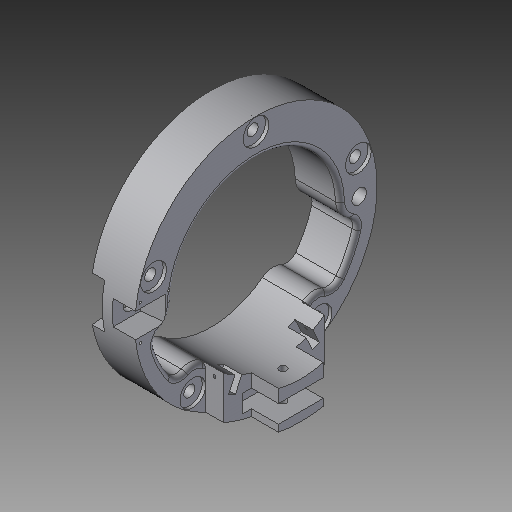
# Autodesk Inventor part: 3218_Coil Holder End_V1
Saved by Autodesk Inventor 2020 (Build 240168000, 168)
## iProperties
Created: 2018-08-02
Part Number: 3218_Coil Holder End_V1
Material: Acetal Resin, White
Document SubType Name: Modeling
Designer: em364
Density: 1.425 g/cm^3
Appearance: Smooth - White
Mass: 120.541 g
Surface Area: 258.548 cm^2
Volume: 84.5901 cm^3
Author: em364
Autodesk Inventor part; units mm, degrees
sketch "Sketch1" plane through (0, 0, 0) normal (1, 0, 0) x (0, 1, 0)
  circle A0 centre (0, 0) radius 54
  circle A1 centre (0, 46) radius 3.25
  circle A2 centre (0, -46) radius 3.25
  circle A3 centre (0, 0) radius 37.5
  circle A4 centre (48, 0) radius 2.5
  circle A5 centre (14.8328, 45.6507) radius 2.5
  circle A6 centre (-38.8328, 28.2137) radius 2.5
  circle A7 centre (-38.8328, -28.2137) radius 2.5
  circle A8 centre (14.8328, -45.6507) radius 2.5
  dimension "d0" = 108
  dimension "d4" = 6.5
  dimension "d5" = 6.5
  dimension "d67" = 75
  dimension "d71" = 0
  dimension "d72" = 0
  dimension "d73" = 46
  dimension "d74" = 46
  dimension "d76" = 5
  dimension "d77" = 48
  dimension "d80" = 360
  constraints: 9 centre point, 11 other
  measures "d0" diameter of A0
  measures "d4" diameter of A2
  measures "d5" diameter of A1
  measures "d67" diameter of A3
  measures "d71" distance of A0.centre A3.centre
  measures "d72" distance of A0.centre A3.centre
  measures "d73" distance of A0.centre A1.centre
  measures "d74" distance of A0.centre A2.centre
  measures "d76" diameter of A4
  measures "d77" distance of A0.centre A4.centre
extrude "Extrusion5" add sketch "Sketch1" along normal blind 20
sketch "Sketch5" plane through (20, 0, 0) normal (1, 0, 0) x (0, 0, -1)
  circle A0 centre (0, 0) radius 37.5 projected
  circle A1 centre (46, 0) radius 3.25 projected
  circle A2 centre (-46, 0) radius 3.25 projected
  circle A3 centre (45.6507, 14.8328) radius 2.5 projected
  circle A4 centre (28.2137, -38.8328) radius 2.5 projected
  circle A5 centre (-28.2137, -38.8328) radius 2.5 projected
  circle A6 centre (-45.6507, 14.8328) radius 2.5 projected
  circle A7 centre (0, 48) radius 2.5 projected
  circle A8 centre (0, 0) radius 54 projected
  circle A9 centre (0, 48) radius 5.75
  circle A10 centre (0, 48) radius 2.5 projected
  circle A11 centre (-45.6507, 14.8328) radius 5.75
  circle A12 centre (-28.2137, -38.8328) radius 5.75
  circle A13 centre (28.2137, -38.8328) radius 5.75
  circle A14 centre (45.6507, 14.8328) radius 5.75
  dimension "d84" = 11.5
  dimension "d87" = 360
  constraints: 5 centre point, 1 coincident, 1 concentric, 11 other
  measures "d84" diameter of A9
extrude "Extrusion6" cut sketch "Sketch5" against normal blind 1.5 contours A9 | A11 | A12 | A13 | A14
sketch "Sketch6" plane through (0, 0, 0) normal (-1, 0, 0) x (0, 0, 1)
  circle A0 centre (0, 0) radius 42 construction
  line L0 (0, 0) -> (20.2657, 62.3715) construction
  circle A1 centre (0, 48) radius 2.5 projected
  line L1 (0, 48) -> (0, 0) construction
  line L2 (10.0924, 40.7694) -> (13.808, 52.2048)
  circle A2 centre (0, 0) radius 54 projected
  line L3 (15.7987, 38.9153) -> (19.5143, 50.3507)
  arc A3 (15.7987, 38.9153) -> (10.0924, 40.7694) centre (0, 0) ccw
  arc A4 (19.5143, 50.3507) -> (13.808, 52.2048) centre (0, 0) ccw
  line L4 (-15.7987, 38.9153) -> (-19.5143, 50.3507)
  line L5 (-10.0924, 40.7694) -> (-13.808, 52.2048)
  arc A5 (-10.0924, 40.7694) -> (-15.7987, 38.9153) centre (0, 0) ccw
  arc A6 (-13.808, 52.2048) -> (-19.5143, 50.3507) centre (0, 0) ccw
  line L6 (-35.6553, 22.1969) -> (-45.3828, 29.2643)
  line L7 (-32.1286, 27.051) -> (-41.8561, 34.1184)
  arc A7 (-32.1286, 27.051) -> (-35.6553, 22.1969) centre (0, 0) ccw
  arc A8 (-41.8561, 34.1184) -> (-45.3828, 29.2643) centre (0, 0) ccw
  line L8 (-41.8927, -3) -> (-53.9166, -3)
  line L9 (-41.8927, 3) -> (-53.9166, 3)
  arc A9 (-41.8927, 3) -> (-41.8927, -3) centre (0, 0) ccw
  arc A10 (-53.9166, 3) -> (-53.9166, -3) centre (0, 0) ccw
  line L10 (-32.1286, -27.051) -> (-41.8561, -34.1184)
  line L11 (-35.6553, -22.1969) -> (-45.3828, -29.2643)
  arc A11 (-35.6553, -22.1969) -> (-32.1286, -27.051) centre (0, 0) ccw
  arc A12 (-45.3828, -29.2643) -> (-41.8561, -34.1184) centre (0, 0) ccw
  line L12 (-10.0924, -40.7694) -> (-13.808, -52.2048)
  line L13 (-15.7987, -38.9153) -> (-19.5143, -50.3507)
  arc A13 (-15.7987, -38.9153) -> (-10.0924, -40.7694) centre (0, 0) ccw
  arc A14 (-19.5143, -50.3507) -> (-13.808, -52.2048) centre (0, 0) ccw
  line L14 (15.7987, -38.9153) -> (19.5143, -50.3507)
  line L15 (10.0924, -40.7694) -> (13.808, -52.2048)
  arc A15 (10.0924, -40.7694) -> (15.7987, -38.9153) centre (0, 0) ccw
  arc A16 (13.808, -52.2048) -> (19.5143, -50.3507) centre (0, 0) ccw
  line L16 (35.6553, -22.1969) -> (45.3828, -29.2643)
  line L17 (32.1286, -27.051) -> (41.8561, -34.1184)
  arc A17 (32.1286, -27.051) -> (35.6553, -22.1969) centre (0, 0) ccw
  arc A18 (41.8561, -34.1184) -> (45.3828, -29.2643) centre (0, 0) ccw
  line L18 (41.8927, 3) -> (53.9166, 3)
  line L19 (41.8927, -3) -> (53.9166, -3)
  arc A19 (41.8927, -3) -> (41.8927, 3) centre (0, 0) ccw
  arc A20 (53.9166, -3) -> (53.9166, 3) centre (0, 0) ccw
  line L20 (32.1286, 27.051) -> (41.8561, 34.1184)
  line L21 (35.6553, 22.1969) -> (45.3828, 29.2643)
  arc A21 (35.6553, 22.1969) -> (32.1286, 27.051) centre (0, 0) ccw
  arc A22 (45.3828, 29.2643) -> (41.8561, 34.1184) centre (0, 0) ccw
  line L22 (-12.9787, 39.9444) -> (0, 0) construction
  line L23 (0, 0) -> (-33.9787, 24.687) construction
  line L24 (0, 0) -> (-33.9787, -24.687) construction
  line L25 (0, 0) -> (-12.9787, -39.9444) construction
  line L26 (0, 0) -> (12.9787, -39.9444) construction
  line L27 (0, 0) -> (33.9787, -24.687) construction
  line L28 (0, 0) -> (33.9787, 24.687) construction
  line L29 (0, 0) -> (59.5549, -8.3699) construction
  line L30 (0, 0) -> (54, 0) construction
  line L31 (41.9025, -2.8595) -> (53.8094, -4.5329)
  line L32 (52.9744, -10.4745) -> (41.0675, -8.8011)
  arc A23 (41.0675, -8.8011) -> (41.9025, -2.8595) centre (0, 0) ccw
  arc A24 (52.9744, -10.4745) -> (53.8094, -4.5329) centre (0, 0) ccw
  line L33 (-41.8927, -3) -> (-53.9166, -3)
  line L34 (-41.9025, -2.8595) -> (-53.8094, -4.5329)
  line L35 (-52.9744, -10.4745) -> (-41.0675, -8.8011)
  arc A25 (-41.9025, -2.8595) -> (-41.0675, -8.8011) centre (0, 0) ccw
  arc A26 (-53.8094, -4.5329) -> (-52.9744, -10.4745) centre (0, 0) ccw
  line L36 (-41.5913, -5.8453) -> (0, 0) construction
  dimension "d91" = 84
  dimension "d92" = 18
  dimension "d93" = 3
  dimension "d94" = 3
  dimension "d97" = 360
  dimension "d99" = 18
  dimension "d100" = 54
  dimension "d101" = 54
  dimension "d102" = 18
  dimension "d103" = 18
  dimension "d104" = 54
  dimension "d105" = 54
  dimension "d106" = 8
  dimension "d107" = 3
  dimension "d108" = 3
  dimension "d109" = 8
  constraints: 74 end point, 65 point on circle, 25 centre point, 15 coincident, 4 parallel, 4 symmetric about line, 1 vertical, 103 other
  measures "d91" diameter of A0
  measures "d92" angle of L0 L1
  measures "d93" distance between parallel lines of L0 L2
  measures "d94" distance between parallel lines of L3 L0
  measures "d99" angle of L22 L1
  measures "d100" angle of L1 L23
  measures "d101" angle of L24 L1
  measures "d102" angle of L1 L25
  measures "d103" angle of L1 L26
  measures "d104" angle of L1 L27
  measures "d105" angle of L1 L28
  measures "d106" angle of L29 L30
  measures "d107" distance between parallel lines of L32 L29
  measures "d108" distance between parallel lines of L29 L31
  measures "d109" angle of L36 L30
extrude "Extrusion7" add sketch "Sketch6" along normal blind 100 contours L2 A2 L3 A3 | L5 A5 L4 A2 | A2 L21 A21 L20 | L7 A7 L6 A2 | L31 L19 A19 | A2 L32 A23 L19 L31 | L34 L8 A25 L35 A2 | L34 A9 L8 | A2 L17 A17 L16 | L11 A11 L10 A2 | A2 L15 A15 L14 | L13 A13 L12 A2
ref_plane "Work Plane4" through (-100, 0, 0) normal (-1, 0, 0) x (0, 0, 1)
sketch "Sketch7" plane through (-100, 0, 0) normal (-1, 0, 0) x (0, 0, 1)
  line L0 (45.3828, 29.2643) -> (35.6553, 22.1969) construction
  arc A0 (35.6553, 22.1969) -> (32.1286, 27.051) centre (0, 0) ccw projected
  line L1 (32.1286, 27.051) -> (41.8561, 34.1184) construction
  arc A1 (41.8561, 34.1184) -> (19.5143, 50.3507) centre (0, 0) ccw projected
  line L2 (19.5143, 50.3507) -> (15.7987, 38.9153) construction
  arc A2 (15.7987, 38.9153) -> (10.0924, 40.7694) centre (0, 0) ccw projected
  line L3 (10.0924, 40.7694) -> (13.808, 52.2048) construction
  arc A3 (13.808, 52.2048) -> (-13.808, 52.2048) centre (0, 0) ccw projected
  line L4 (-13.808, 52.2048) -> (-10.0924, 40.7694) construction
  arc A4 (-10.0924, 40.7694) -> (-15.7987, 38.9153) centre (0, 0) ccw projected
  line L5 (-15.7987, 38.9153) -> (-19.5143, 50.3507) construction
  arc A5 (-19.5143, 50.3507) -> (-41.8561, 34.1184) centre (0, 0) ccw projected
  line L6 (-41.8561, 34.1184) -> (-32.1286, 27.051) construction
  arc A6 (-32.1286, 27.051) -> (-35.6553, 22.1969) centre (0, 0) ccw projected
  line L7 (-35.6553, 22.1969) -> (-45.3828, 29.2643) construction
  arc A7 (-45.3828, 29.2643) -> (-53.8094, -4.5329) centre (0, 0) ccw projected
  line L8 (-53.8094, -4.5329) -> (-41.9025, -2.8595) construction
  arc A8 (-41.9025, -2.8595) -> (-41.0675, -8.8011) centre (0, 0) ccw projected
  line L9 (-41.0675, -8.8011) -> (-52.9744, -10.4745) construction
  arc A9 (-52.9744, -10.4745) -> (-45.3828, -29.2643) centre (0, 0) ccw projected
  line L10 (-45.3828, -29.2643) -> (-35.6553, -22.1969) construction
  arc A10 (-35.6553, -22.1969) -> (-32.1286, -27.051) centre (0, 0) ccw projected
  line L11 (-32.1286, -27.051) -> (-41.8561, -34.1184) construction
  arc A11 (-41.8561, -34.1184) -> (-19.5143, -50.3507) centre (0, 0) ccw projected
  line L12 (-19.5143, -50.3507) -> (-15.7987, -38.9153) construction
  arc A12 (-15.7987, -38.9153) -> (-10.0924, -40.7694) centre (0, 0) ccw projected
  line L13 (-10.0924, -40.7694) -> (-13.808, -52.2048) construction
  arc A13 (-13.808, -52.2048) -> (13.808, -52.2048) centre (0, 0) ccw projected
  line L14 (13.808, -52.2048) -> (10.0924, -40.7694) construction
  arc A14 (10.0924, -40.7694) -> (15.7987, -38.9153) centre (0, 0) ccw projected
  line L15 (15.7987, -38.9153) -> (19.5143, -50.3507) construction
  arc A15 (19.5143, -50.3507) -> (41.8561, -34.1184) centre (0, 0) ccw projected
  line L16 (41.8561, -34.1184) -> (32.1286, -27.051) construction
  arc A16 (32.1286, -27.051) -> (35.6553, -22.1969) centre (0, 0) ccw projected
  line L17 (35.6553, -22.1969) -> (45.3828, -29.2643) construction
  arc A17 (45.3828, -29.2643) -> (52.9744, -10.4745) centre (0, 0) ccw projected
  line L18 (52.9744, -10.4745) -> (41.0675, -8.8011) construction
  arc A18 (41.0675, -8.8011) -> (41.9025, -2.8595) centre (0, 0) ccw projected
  line L19 (41.9025, -2.8595) -> (53.8094, -4.5329) construction
  arc A19 (53.8094, -4.5329) -> (45.3828, 29.2643) centre (0, 0) ccw projected
  circle A20 centre (0, 48) radius 2.5 construction
  circle A21 centre (45.6507, 14.8328) radius 2.5 construction
  circle A22 centre (28.2137, -38.8328) radius 2.5 construction
  circle A23 centre (-28.2137, -38.8328) radius 2.5 construction
  circle A24 centre (-45.6507, 14.8328) radius 2.5 construction
  circle A25 centre (46, 0) radius 3.25 construction
  circle A26 centre (-46, 0) radius 3.25 projected
  circle A27 centre (0, 0) radius 37.5 projected
  circle A28 centre (0, 0) radius 54
  circle A29 centre (0, 0) radius 37.5 projected
  line L20 (0, 0) -> (0, -54) construction
  circle A30 centre (0, 0) radius 54 projected
  line L21 (0, 0) -> (-32.0095, -68.6446) construction
  circle A31 centre (0, 0) radius 42 construction
  line L22 (0, 0) -> (32.0095, -68.6446) construction
  line L23 (0, 0) -> (-46, 0) construction
  line L24 (0, 0) -> (-32.0095, 68.6446) construction
  line L25 (0, 0) -> (32.0095, 68.6446) construction
  arc A32 (-21.9138, 30.4308) -> (-21.9138, -30.4308) centre (0, 0) ccw
  arc A33 (9.2255, 36.3475) -> (-9.2255, 36.3475) centre (0, 0) ccw
  arc A34 (21.9138, -30.4308) -> (21.9138, 30.4308) centre (0, 0) ccw
  arc A35 (-9.2255, -36.3475) -> (9.2255, -36.3475) centre (0, 0) ccw
  circle A36 centre (0, 0) radius 37.5
  dimension "d113" = 25
  dimension "d115" = 84
  dimension "d120" = 25
  dimension "d123" = 25
  dimension "d124" = 25
  constraints: 12 end point, 11 point on circle, 9 symmetric about line, 7 centre point, 5 coincident, 1 concentric, 1 horizontal, 2 other
  measures "d113" angle of L21 L20
  measures "d115" diameter of A31
  measures "d120" angle of L20 L22
  measures "d123" angle of L20 L24
  measures "d124" angle of L20 L25
extrude "Extrusion12" add sketch "Sketch7" along normal blind 10
sketch "Sketch11" plane through (-110, 0, 0) normal (-1, 0, 0) x (0, 0, 1)
  circle A0 centre (0, 0) radius 37.5 projected
  circle A1 centre (-46, 0) radius 3.25 projected
  circle A2 centre (0, 0) radius 54 projected
  circle A3 centre (0, 0) radius 42 construction
  line L0 (0, 0) -> (-19.8631, 42.5965) construction
  arc A4 (-13.2974, 45.0797) -> (-25.9857, 39.1631) centre (0, 0) ccw projected
  line L1 (0, 0) -> (19.8631, 42.5965) construction
  arc A5 (25.9857, 39.1631) -> (13.2974, 45.0797) centre (0, 0) ccw projected
  line L2 (0, 0) -> (19.8631, -42.5965) construction
  arc A6 (13.2974, -45.0797) -> (25.9857, -39.1631) centre (0, 0) ccw projected
  arc A7 (37.5, 0) -> (37.5, 0) centre (0, 0) ccw projected
  line L3 (0, 0) -> (-19.8631, -42.5965) construction
  arc A8 (-25.9857, -39.1631) -> (-13.2974, -45.0797) centre (0, 0) ccw projected
  circle A9 centre (-17.75, 38.0649) radius 1.7
  circle A10 centre (17.75, 38.0649) radius 1.7
  circle A11 centre (17.75, -38.0649) radius 1.7
  circle A12 centre (-17.75, -38.0649) radius 1.7
  dimension "d151" = 84
  dimension "d152" = 3.4
  dimension "d153" = 3.4
  dimension "d154" = 3.4
  dimension "d155" = 3.4
  constraints: 8 end point, 8 point on circle, 5 centre point, 4 point on line, 1 coincident
  measures "d151" diameter of A3
  measures "d152" diameter of A9
  measures "d153" diameter of A10
  measures "d154" diameter of A11
  measures "d155" diameter of A12
extrude "Extrusion14" cut sketch "Sketch11" against normal blind 10 contours A9 | A10 | A11 | A12
ref_plane "Work Plane5" through (-50, 0, 0) normal (1, 0, 0) x (0, 0, -1)
sketch "Sketch12" plane through (-50, 0, 0) normal (1, 0, 0) x (0, 0, -1)
  circle A0 centre (45.6507, 14.8328) radius 5.75 construction
  circle A1 centre (-28.2137, -38.8328) radius 5.75 construction
  circle A2 centre (0, 48) radius 5.75 construction
  circle A3 centre (-45.6507, 14.8328) radius 5.75 construction
  circle A4 centre (28.2137, -38.8328) radius 5.75 construction
  circle A5 centre (0, 0) radius 37.5 projected
  circle A6 centre (46, 0) radius 3.25 projected
  circle A7 centre (-46, 0) radius 3.25 construction
  circle A8 centre (0, 0) radius 54 projected
extrude "Extrusion15" add sketch "Sketch12" along normal mid plane 6
sketch "Sketch13" plane through (20, 0, 0) normal (1, 0, 0) x (0, 0, -1)
  circle A0 centre (0, 0) radius 54 construction
  circle A1 centre (0, 0) radius 37.5 construction
  line L0 (0, 0) -> (0, -37.5)
  line L1 (0, 0) -> (60.8881, 0) construction
  line L2 (-22.5, -30) -> (-22.5, -49.0892)
  line L3 (22.5, -30) -> (22.5, -49.0892)
  arc A2 (-22.5, -30) -> (22.5, -30) centre (0, 0) ccw
  arc A3 (-22.5, -49.0892) -> (22.5, -49.0892) centre (0, 0) ccw
  dimension "d166" = 22.5
  dimension "d167" = 22.5
  constraints: 8 end point, 6 point on circle, 2 centre point, 2 coincident, 2 symmetric about line, 2 vertical, 1 horizontal, 2 other
  measures "d166" distance between parallel lines of L2 L0
  measures "d167" distance between parallel lines of L3 L0
extrude "Extrusion16" add sketch "Sketch13" along normal blind 8
sketch "Sketch14" plane through (28, 0, 0) normal (1, 0, 0) x (0, 0, -1)
  arc A0 (-22.5, -30) -> (22.5, -30) centre (0, 0) ccw projected
  line L0 (0, 0) -> (0, -37.5)
  circle A1 centre (0, 0) radius 54 projected
  line L1 (12, -42) -> (-12, -42) construction
  line L2 (-10, -42) -> (-10, -36.1421)
  line L3 (10, -42) -> (10, -36.1421)
  arc A2 (-10, -36.1421) -> (10, -36.1421) centre (0, 0) ccw
  line L4 (-10, -42) -> (10, -42)
  line L5 (-10, -50) -> (-10, -53.066)
  line L6 (10, -50) -> (10, -53.066)
  line L7 (-10, -50) -> (10, -50)
  arc A3 (-10, -53.066) -> (10, -53.066) centre (0, 0) ccw
  dimension "d174" = 16.5
  dimension "d194" = 10
  dimension "d195" = 10
  dimension "d196" = 8
  dimension "d197" = 10
  dimension "d198" = 10
  dimension "d211" = 50
  constraints: 16 end point, 5 point on circle, 4 symmetric about line, 2 centre point, 2 collinear, 1 coincident, 1 perpendicular, 1 point on line, 1 vertical
  measures "d174" radial gap between concentric circles of A1 A0
  measures "d194" distance between parallel lines of L0 L2
  measures "d195" distance between parallel lines of L0 L5
  measures "d196" distance between parallel lines of L7 L4
  measures "d197" distance between parallel lines of L0 L3
  measures "d198" distance between parallel lines of L0 L6
  measures "d211" distance from line of L7 point (0, 0)
extrude "Extrusion17" add sketch "Sketch14" along normal blind 12 contours A0 L3 L4 L2 | L5 L7 L6 A1 picked at (-1.1168, -51.2987)
sketch "Sketch16" plane through (28, 0, 0) normal (1, 0, 0) x (0, 0, -1)
  arc A0 (22.5, -49.0892) -> (-22.5, -49.0892) centre (0, 0) ccw projected
  line L0 (0, 0) -> (0, 37.5)
  circle A1 centre (0, 0) radius 37.5 construction
  line L1 (0, 0) -> (-18.722, -40.1494) construction
  line L2 (-18.722, -40.1494) -> (-17.1813, -40.8679)
  line L3 (-17.1813, -40.8679) -> (-14.2912, -34.6701)
  line L4 (-18.722, -40.1494) -> (-20.2627, -39.431)
  line L5 (-20.2627, -39.431) -> (-17.3726, -33.2331)
  line L6 (0, 0) -> (18.722, -40.1494) construction
  line L7 (18.722, -40.1494) -> (17.1813, -40.8679)
  line L8 (17.1813, -40.8679) -> (14.2912, -34.6701)
  line L9 (20.2627, -39.431) -> (17.3726, -33.2331)
  line L10 (18.722, -40.1494) -> (20.2627, -39.431)
  arc A2 (-17.3726, -33.2331) -> (-14.2912, -34.6701) centre (0, 0) ccw
  arc A3 (14.2912, -34.6701) -> (17.3726, -33.2331) centre (0, 0) ccw
  dimension "d187" = 25
  dimension "d188" = 44.3
  dimension "d190" = 1.7
  dimension "d212" = 44.3
  constraints: 22 end point, 7 symmetric about line, 6 point on circle, 2 centre point, 2 coincident, 2 perpendicular
  measures "d187" angle of L0 L1
  measures "d188" distance of L0.start L1.end
  measures "d190" distance of L1.end L2.end
  measures "d212" distance from line of L10 point (0, 0)
extrude "Extrusion19" cut sketch "Sketch16" against normal blind 8
ref_plane "Work Plane7" through (28, -32, -10) normal (0, -1, 0) x (1, 0, 0)
sketch "Sketch18" plane through (28, -32, -10) normal (0, -1, 0) x (1, 0, 0)
  line L0 (0, 20) -> (12, 20) construction
  line L1 (0, 0) -> (0, 20) construction
  line L2 (0, 0) -> (12, 0) construction
  line L3 (12, 20) -> (12, 0) construction
  circle A0 centre (4, 10) radius 1.65
  point P0 (-28, 10)
  dimension "d200" = 3.3
  dimension "d201" = 10
  dimension "d202" = 8
  dimension "d203" = 20
  constraints: 1 centre point
  measures "d200" diameter of A0
  measures "d201" distance from line of L0 A0.centre
  measures "d202" distance from line of A0.centre L3
  measures "d203" distance of L0.end L2.end
extrude "Extrusion20" cut sketch "Sketch18" along normal through all
sketch "Sketch19" plane through (-110, 0, 0) normal (-1, 0, 0) x (0, 0, 1)
  circle A0 centre (0, 0) radius 54 construction
  circle A1 centre (0, 0) radius 50 construction
  line L0 (-6.3, 50) -> (-6.3, 53.6312)
  arc A2 (13.808, 52.2048) -> (-13.808, 52.2048) centre (0, 0) ccw projected
  line L1 (0, 0) -> (0, 50) construction
  line L2 (0, 50) -> (6.1226, 50) construction
  line L3 (6.3, 50) -> (6.3, 53.6312)
  line L4 (0, 50) -> (-1.1865, 50) construction
  arc A3 (-6.3, 50) -> (6.3, 50) centre (0, 50) ccw
  circle A4 centre (0, 0) radius 54
  dimension "d206" = 100
  dimension "d208" = 50
  dimension "d213" = 6.3
  dimension "d215" = 0
  constraints: 10 end point, 6 point on circle, 3 coincident, 2 centre point, 2 horizontal, 2 vertical, 1 parallel, 1 point on line, 3 other
  measures "d206" diameter of A1
  measures "d208" distance of A1.centre L1.end
  measures "d213" radius of A3
  measures "d215" distance from line of L1 L4.start
extrude "Extrusion21" cut sketch "Sketch19" against normal up to surface (63 mm away) contours L0 A2 L3 A3
sketch "Sketch20" plane through (0, 0, 0) normal (-1, 0, 0) x (0, 0, 1)
  circle A0 centre (0, 0) radius 54
  constraints: 1 centre point, 1 coincident
extrude "Extrusion22" cut sketch "Sketch20" along normal through all
sketch "Sketch21" plane through (28, 0, 0) normal (1, 0, 0) x (0, 0, -1)
  line L0 (-14, -42) -> (14, -42)
  line L1 (14, -42) -> (14, -50)
  line L2 (14, -50) -> (-14, -50)
  line L3 (-14, -50) -> (-14, -42)
  line L4 (-10, -36.1421) -> (-10, -42) projected
  line L5 (10, -42) -> (10, -36.1421) projected
  line L6 (1.65, -42) -> (-1.65, -42) projected
  point P0 (0, 0)
  point P1 (0, -42)
  dimension "d218" = 8
  dimension "d219" = 28
  dimension "d220" = 20
  dimension "d221" = 14
  constraints: 8 end point, 2 parallel, 1 horizontal, 1 midpoint, 1 perpendicular
  measures "d218" distance of L0.end L1.end
  measures "d219" distance of L0.start L0.end
  measures "d220" distance between parallel lines of L4 L5
  measures "d221" distance from line of L3 point (0, -42)
extrude "Extrusion23" cut sketch "Sketch21" against normal blind 5
fillet "Fillet2" radius 3 2 edges at (23, -46, 14) (23, -46, -14)
ref_plane "Work Plane8" through (28, -35.2048, 29.3258) normal (0, -0.4226183, -0.9063078) x (-1, 0, 0)
sketch "Sketch23" plane through (28, -35.2048, 29.3258) normal (0, -0.4226183, -0.9063078) x (-1, 0, 0)
  circle A0 centre (4, 4.6019) radius 0.6
  line L0 (0, 7.6019) -> (0, -9.6988) projected
  line L1 (8, 0.1813) -> (8, 7.6019) projected
  line L2 (8, 7.6019) -> (0, 7.6019) projected
  point P0 (28, 44.3)
  dimension "d226" = 1.2
  dimension "d227" = 4
  dimension "d228" = 8
  dimension "d229" = 3
  constraints: 1 centre point
  measures "d226" diameter of A0
  measures "d227" distance from line of A0.centre L0
  measures "d228" distance between parallel lines of L0 L1
  measures "d229" distance from line of L2 A0.centre
extrude "Extrusion24" cut sketch "Sketch23" along normal up to surface (13.4 mm away)
mirror "Mirror1" about plane through (0, 0, 0) normal (0, 0, 1) of "Extrusion24"
sketch "Sketch24" plane through (0, 0, 0) normal (-1, 0, 0) x (0, 0, 1)
  circle A0 centre (0, 48) radius 2.5 projected
  line L0 (4.5, 50.5981) -> (4.5, 45.4019)
  line L1 (4.5, 45.4019) -> (0, 42.8038)
  line L2 (0, 42.8038) -> (-4.5, 45.4019)
  line L3 (-4.5, 45.4019) -> (-4.5, 50.5981)
  line L4 (-4.5, 50.5981) -> (0, 53.1962)
  line L5 (0, 53.1962) -> (4.5, 50.5981)
  line L6 (0, 75.6003) -> (0, -75.6017) projected
  point P0 (0, 0)
  dimension "d232" = 9
  dimension "d233" = 0
  constraints: 12 end point, 1 coincident, 13 other
  measures "d232" distance between parallel lines of L2 L5
  measures "d233" distance from line of L6 L4.end
extrude "Extrusion25" cut sketch "Sketch24" against normal blind 4 contours A0 L6 L5 L0 L1 | A0 L6 L2 L3 L4
pattern_circular "Circular Pattern1" count 5 over 360 about axis through (0, 0, 0) along (1, 0, 0) of "Extrusion25"
sketch "Sketch27" plane through (20, 0, 0) normal (1, 0, 0) x (0, 0, -1)
  line L0 (-40.5, 5.5) -> (-54, 5.5)
  line L1 (-54, 5.5) -> (-54, -5.5)
  line L2 (-54, -5.5) -> (-40.5, -5.5)
  line L3 (-40.5, -5.5) -> (-40.5, 5.5)
  arc A0 (22.5, -49.0892) -> (-22.5, -49.0892) centre (0, 0) ccw projected
  circle A1 centre (-46, 0) radius 3.25 projected
  circle A2 centre (-46, 0) radius 5.5
  dimension "d245" = 11
  constraints: 8 end point, 4 tangent, 2 parallel, 1 centre point, 1 coincident, 1 horizontal, 1 perpendicular
  measures "d245" diameter of A2
extrude "Extrusion27" cut sketch "Sketch27" against normal blind 10 contours L3 A2 L0 | A2 L2 A0 L0 | A2 | L3 L2 A2 | A0 L1 L0 | A0 L2 L1 | A1
sketch "Sketch28" plane through (20, 5.5, 40.5) normal (0, -1, 0) x (1, 0, 0)
  line L0 (0, 0) -> (-10, 0) projected
  line L1 (-10, 0) -> (-10, 0.8749)
  line L2 (-10, 13.2192) -> (-10, 0) projected
  line L3 (0, 0) -> (-10, 0.8749)
  line L4 (-10, 0) -> (0, 0)
  point P0 (-20, -40.5)
  dimension "d246" = 5
  constraints: 6 end point, 1 perpendicular, 1 point on line
  measures "d246" angle of L0 L3
extrude "Extrusion28" add sketch "Sketch28" along normal up to surface (11 mm away)
sketch "Sketch29" plane through (0, 0, 0) normal (-1, 0, 0) x (0, 0, 1)
  circle A0 centre (0, 0) radius 54 projected
  line L0 (53.066, -10) -> (36.6367, -8)
  circle A1 centre (0, 0) radius 37.5 projected
  circle A2 centre (46, 0) radius 3.25 projected
  line L1 (49.25, 0) -> (42.75, 0)
  line L2 (53.066, 10) -> (36.6367, 8)
  arc A3 (53.066, -10) -> (53.066, 10) centre (0, 0) ccw
  arc A4 (36.6367, -8) -> (36.6367, 8) centre (0, 0) ccw
  dimension "d249" = 10
  dimension "d250" = 8
  constraints: 6 end point, 6 point on circle, 2 centre point, 2 symmetric about line, 1 horizontal, 6 other
  measures "d249" vertical distance of point (0, 0) L0.start
  measures "d250" vertical distance of point (0, 0) L0.end
extrude "Extrusion29" cut sketch "Sketch29" against normal blind 5.5 contours A0 L0 A1 L2 picked at (45.1037, -7.0754)
sketch "Sketch30" plane through (5.5, 0, 0) normal (-1, 0, 0) x (0, 0, 1)
  circle A0 centre (46, 0) radius 3.25 projected
  circle A1 centre (46, 0) radius 5.5
  point P0 (0, 0)
  dimension "d253" = 11
  constraints: 1 centre point, 1 coincident
  measures "d253" diameter of A1
extrude "Extrusion30" cut sketch "Sketch30" against normal blind 2
sketch "Sketch31" plane through (5.5, 0, 0) normal (-1, 0, 0) x (0, 0, 1)
  circle A0 centre (0, 0) radius 52.2
  circle A1 centre (51.6127, 7.8083) radius 0.6
  line L0 (36.6367, 8) -> (53.066, 10) projected
  circle A2 centre (38.8001, 6.2486) radius 0.6
  circle A3 centre (46, 0) radius 5.5 projected
  line L1 (51.5, 0) -> (40.4184, 0)
  circle A4 centre (51.6127, -7.8083) radius 0.6
  dimension "d257" = 104.4
  dimension "d258" = 1.2
  dimension "d259" = 2
  dimension "d260" = 1.2
  dimension "d261" = 2
  constraints: 3 centre point, 2 end point, 1 horizontal, 1 horizontal alignment, 1 symmetric about line, 5 other
  measures "d258" diameter of A1
  measures "d259" distance from line of L0 A1.centre
  measures "d260" diameter of A2
  measures "d261" distance from line of L0 A2.centre
extrude "Extrusion31" cut sketch "Sketch31" against normal through all contours A1 A0 | A0 A1 | A4 A0 | A0 A4 | A2
sketch "Sketch32" plane through (20, 0, 0) normal (1, 0, 0) x (0, 0, -1)
  circle A0 centre (-38.8001, -6.2486) radius 0.6 projected
  line L0 (0, 0) -> (-38.8001, -6.2486) construction
  line L1 (-38.8001, -6.2486) -> (-53.3131, -8.5858) construction
  arc A1 (-53.7192, -5.5) -> (-22.5, -49.0892) centre (0, 0) ccw construction
  line L2 (0, 0) -> (-39.4931, -36.8279) construction
  line L3 (0, 0) -> (54, 0) construction
  arc A2 (-36.6367, 8) -> (-36.6367, -8) centre (0, 0) ccw projected
  arc A3 (-37.023, -5.9624) -> (-27.4258, -25.5749) centre (0, 0) ccw
  arc A4 (-46.0566, -7.4172) -> (-34.1177, -31.8152) centre (0, 0) ccw
  line L4 (-46.0566, -7.4172) -> (-37.023, -5.9624)
  line L5 (-27.4258, -25.5749) -> (-34.1177, -31.8152)
  line L6 (0, 0) -> (0, -37.5)
  arc A5 (-36.6367, -8) -> (-36.6367, 8) centre (0, 0) ccw projected
  arc A6 (27.4258, -25.5749) -> (37.023, -5.9624) centre (0, 0) ccw
  arc A7 (34.1177, -31.8152) -> (46.0566, -7.4172) centre (0, 0) ccw
  line L7 (46.0566, -7.4172) -> (37.023, -5.9624)
  line L8 (27.4258, -25.5749) -> (34.1177, -31.8152)
  dimension "d264" = 137
  constraints: 18 end point, 12 point on circle, 4 centre point, 4 point on line, 4 symmetric about line, 2 coincident, 2 collinear, 1 equal length, 1 horizontal, 1 midpoint, 1 vertical, 2 other
  measures "d264" angle of L2 L3
extrude "Extrusion32" cut sketch "Sketch32" against normal through all contours A0 L4 | A0 L4 A2 A3 L5 A4 | L7 A7 L8 A5 picked at (-38.8337, -6.4458)
fillet "Fillet3" radius 5 4 edges at (12.75, -7.4172, 46.0566) (10, -31.8152, 34.1177) (10, -31.8152, -34.1177) (10, -7.4172, -46.0566)
fillet "Fillet4" radius 8 2 edges at (10, -25.5749, 27.4258) (10, -25.5749, -27.4258)
fillet "Fillet5" radius 10 2 edges at (12.75, -5.9624, 37.023) (10, -5.9624, -37.023)
fillet "Fillet6" radius 2 19 edges at (20, -3.2886, -38.7022) (20, -6.9596, -42.1585) (20, -9.6302, -44.6607) (20, -20.5044, -41.9022) (20, -29.4086, -34.8023) (20, -28.1642, -26.6797) (20, -28.8534, -31.087) (20, -29.8765, -22.6637) (20, -3.2886, 38.7022) (20, -6.9596, 42.1585) (20, -7.9371, 43.5248) (20, -10.8594, 44.9852) (20, -20.5044, 41.9022) (20, -29.4086, 34.8023) (20, -28.1642, 26.6797) (20, -28.8534, 31.087) (20, -29.8765, 22.6637) (20, 26.9345, -26.0918) (20, 26.9345, 26.0918)
equation "\"d195\" = d194"
body "Solid2"
